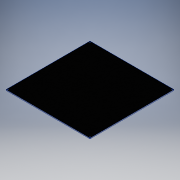
# Autodesk Inventor part: Heated Bed
Saved by Autodesk Inventor 2016 (Build 200138000, 138)
## iProperties
Created: 2017-02-12
Part Number: Heated Bed
Material: Aluminum 6061
Document SubType Name: Modeling
Designer: Scott
Density: 2.7 g/cm^3
Appearance: Aluminum - Flat
Author: Scott
Autodesk Inventor part; units mm, degrees
ref_plane "YZ Plane" through (0, 0, 0) normal (1, 0, 0) x (0, 1, 0)
sketch "Sketch1" plane through (0, 0, 0) normal (0, 0, 1) x (1, 0, 0)
  line L0 (0, 0) -> (338.7718, 0) construction
  line L1 (0, 0) -> (0, 234.489) construction
  line L2 (-107, 107) -> (107, 107)
  line L3 (107, 107) -> (107, -107)
  line L4 (107, -107) -> (-107, -107)
  line L5 (-107, -107) -> (-107, 107)
  point P0 (107, 0)
  point P1 (0, 107)
  dimension "d0" = 214
  dimension "d1" = 214
  constraints: 12 end point, 2 horizontal, 2 midpoint, 2 parallel, 2 point on line, 1 perpendicular, 1 vertical
  measures "d0" distance of L2.start L2.end
  measures "d1" distance of L2.end L3.end
extrude "Extrusion1" add sketch "Sketch1" along normal blind 3
sketch "Sketch2" plane through (0, 0, 0) normal (0, 0, -1) x (-1, 0, 0)
  line L0 (0, 0) -> (359.3191, 0) construction
  line L1 (0, 0) -> (0, 231.2713) construction
  line L2 (-105, 105) -> (105, 105) construction
  line L3 (105, 105) -> (105, -105) construction
  line L4 (105, -105) -> (-105, -105) construction
  line L5 (-105, -105) -> (-105, 105) construction
  point P0 (0, 105)
  point P1 (105, 0)
  dimension "d4" = 210
  dimension "d5" = 210
  constraints: 12 end point, 4 coincident, 2 horizontal, 2 midpoint, 2 parallel, 2 point on line, 1 perpendicular, 1 vertical
  measures "d4" distance of L2.start L2.end
  measures "d5" distance of L2.end L3.end
hole "Hole1" at (105, 105, 0) at (-105, 105, 0) at (-105, -105, 0) at (105, -105, 0) direction (0, 0, 1) diameter 3 end through all
fillet "Fillet1" radius 0.5 4 edges at (107, 107, 1.5) (-107, 107, 1.5) (-107, -107, 1.5) (107, -107, 1.5)
ref_plane "Work Plane1" through (0, -106.5, 0) normal (-1, 0, 0) x (0, 0, 1)
ref_plane "Work Plane2" through (-106.5, 0, 0) normal (0, -1, 0) x (1, 0, 0)
equation "\"d0\" = platform_width"
equation "\"d1\" = platform_depth"
equation "\"d4\" = hole_spacing_width"
equation "\"d5\" = hole_spacing_depth"
equation "\"platform_width\" = 214"
equation "\"platform_depth\" = 214"
equation "\"hole_spacing_width\" = 210"
equation "\"hole_spacing_depth\" = 210"
equation "\"d14\" = -0.5 * platform_width"
equation "\"d15\" = -0.5 * platform_depth"
equation "\"bed_cl_y_offset\" = 173.25"
body "Solid1"
